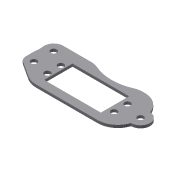
# Autodesk Inventor part: Adapter
Saved by Autodesk Inventor 2015 (Build 190159000, 159)
## iProperties
Created: 2015-02-12
Part Number: Adapter
Material: Generisch
Document SubType Name: Modeling
Designer: Luki
Density: 1 g/cm^3
Appearance: Vorgabe
Author: Luki
Autodesk Inventor part; units mm, degrees
ref_plane "YZ Plane" through (0, 0, 0) normal (1, 0, 0) x (0, 1, 0)
ref_plane "XZ Plane" through (0, 0, 0) normal (0, 1, 0) x (-1, 0, 0)
ref_plane "XY Plane" through (0, 0, 0) normal (0, 0, 1) x (1, 0, 0)
sketch "Skizze1" plane through (0, 0, 0) normal (0, 0, 1) x (1, 0, 0)
  line L0 (0, 78) -> (0, -13) projected
  line L1 (-15, 0) -> (90, 0) projected
  line L2 (0, 0) -> (75, 0)
  line L3 (75, 0) -> (75, 35)
  line L4 (75, 35) -> (0, 35)
  line L5 (0, 35) -> (0, 0)
  arc A0 (24, 35) -> (56, 35) centre (40, 65) ccw
  dimension "d0" = 75
  dimension "d1" = 35
  dimension "d3" = 35
  dimension "d4" = 30
  dimension "d6" = 34
  constraints: 8 end point, 2 parallel, 2 point on circle, 2 point on line, 1 centre point, 1 horizontal, 1 perpendicular
  measures "d0" distance between parallel lines of L3 L0
  measures "d1" distance between parallel lines of L4 L1
  measures "d3" distance from line of L3 A0.centre
  measures "d4" distance from line of L4 A0.centre
  measures "d6" radius of A0
extrude "Extrusion1" add sketch "Skizze1" along normal blind 2 contours L4 A0 L3 L1 L0
sketch "Skizze2" plane through (0, 0, 2) normal (0, 0, 1) x (1, 0, 0)
  line L0 (36, 6) -> (57, 6)
  line L1 (57, 6) -> (57, 27)
  line L2 (57, 27) -> (36, 27)
  line L3 (36, 27) -> (36, 6)
  line L4 (36, 6) -> (57, 27) construction
  line L5 (57, 6) -> (36, 27) construction
  line L6 (57, 27) -> (15, 27)
  line L7 (15, 27) -> (15, 6)
  line L8 (15, 6) -> (57, 6)
  line L9 (57, 6) -> (57, 27)
  line L10 (75, 0) -> (75, 35) projected
  line L11 (24, 35) -> (0, 35) projected
  circle A0 centre (61.35, 21.5) radius 2.25
  circle A1 centre (61.35, 11.5) radius 2.25
  circle A2 centre (11.85, 11.5) radius 2.25
  circle A3 centre (11.85, 21.5) radius 2.25
  point P0 (0, 0)
  point P1 (46.5, 16.5)
  dimension "d9" = 21
  dimension "d10" = 21
  dimension "d11" = 42
  dimension "d12" = 0
  dimension "d13" = 18
  dimension "d14" = 8
  dimension "d15" = 4.5
  dimension "d16" = 4.5
  dimension "d17" = 4.5
  dimension "d18" = 4.5
  dimension "d19" = 14.85
  dimension "d20" = 5
  dimension "d21" = 5
  dimension "d22" = 14.85
  dimension "d23" = 34.65
  dimension "d24" = 34.65
  dimension "d27" = 5
  dimension "d28" = 5
  constraints: 20 end point, 4 centre point, 4 parallel, 2 horizontal, 2 midpoint, 2 perpendicular
  measures "d9" distance between parallel lines of L0 L2
  measures "d10" distance between parallel lines of L3 L1
  measures "d11" distance between parallel lines of L1 L7
  measures "d12" distance between parallel lines of L0 L8
  measures "d13" distance between parallel lines of L10 L1
  measures "d14" distance between parallel lines of L11 L6
  measures "d15" diameter of A0
  measures "d16" diameter of A1
  measures "d17" diameter of A3
  measures "d18" diameter of A2
  measures "d19" horizontal distance of point (46.5, 16.5) A1.centre
  measures "d20" vertical distance of point (46.5, 16.5) A1.centre
  measures "d21" vertical distance of point (46.5, 16.5) A0.centre
  measures "d22" horizontal distance of point (46.5, 16.5) A0.centre
  measures "d23" horizontal distance of point (46.5, 16.5) A3.centre
  measures "d24" horizontal distance of point (46.5, 16.5) A2.centre
  measures "d27" vertical distance of point (46.5, 16.5) A2.centre
  measures "d28" vertical distance of point (46.5, 16.5) A3.centre
extrude "Extrusion2" cut sketch "Skizze2" against normal blind 2
sketch "Skizze3" plane through (0, 0, 2) normal (0, 0, 1) x (1, 0, 0)
  circle A0 centre (11.85, 21.5) radius 2.25 projected
  circle A1 centre (61.35, 11.5) radius 2.25 projected
  circle A2 centre (61.35, 21.5) radius 2.25 projected
  circle A3 centre (11.85, 11.5) radius 2.25 projected
  line L0 (15, 27) -> (15, 6) projected
  line L1 (15, 6) -> (57, 6) projected
  line L2 (57, 6) -> (57, 27) projected
  line L3 (57, 27) -> (15, 27) projected
  line L4 (0, 0) -> (0, 35) projected
  line L5 (0, 35) -> (24, 35) projected
  arc A4 (24, 35) -> (56, 35) centre (40, 65) ccw projected
  line L6 (56, 35) -> (75, 35) projected
  line L7 (75, 35) -> (75, 0) projected
  line L8 (75, 0) -> (0, 0) projected
  line L9 (75, 0) -> (75, 35) projected
  circle A5 centre (75, 17.5) radius 7
  line L10 (75, 0) -> (75, 35) projected
  dimension "d31" = 14
  dimension "d32" = 35
  dimension "d33" = 17.5
  constraints: 2 midpoint, 1 centre point
  measures "d31" diameter of A5
  measures "d32" distance between parallel lines of L8 L6
  measures "d33" distance from line of L8 A5.centre
extrude "Extrusion3" add sketch "Skizze3" against normal blind 2 contours A5 L7 | L7 A5
sketch "Skizze4" plane through (0, 0, 2) normal (0, 0, 1) x (1, 0, 0)
  circle A0 centre (11.85, 21.5) radius 2.25 projected
  circle A1 centre (61.35, 11.5) radius 2.25 projected
  circle A2 centre (61.35, 21.5) radius 2.25 projected
  circle A3 centre (11.85, 11.5) radius 2.25 projected
  line L0 (15, 27) -> (15, 6) projected
  line L1 (15, 6) -> (57, 6) projected
  line L2 (57, 6) -> (57, 27) projected
  line L3 (57, 27) -> (15, 27) projected
  line L4 (0, 0) -> (0, 35) projected
  line L5 (0, 35) -> (24, 35) projected
  arc A4 (24, 35) -> (56, 35) centre (40, 65) ccw projected
  line L6 (56, 35) -> (75, 35) projected
  line L7 (75, 35) -> (75, 24.5) projected
  arc A5 (75, 10.5) -> (75, 24.5) centre (75, 17.5) ccw projected
  line L8 (75, 10.5) -> (75, 0) projected
  line L9 (75, 0) -> (0, 0) projected
  circle A6 centre (75, 17.5) radius 2.25
  dimension "d36" = 4.5
  constraints: 1 centre point, 1 coincident
  measures "d36" diameter of A6
extrude "Extrusion4" cut sketch "Skizze4" against normal blind 2 contours A6
fillet "Rundung1" radius 15 1 edges at (0, 0, 1)
sketch "Skizze5" plane through (0, 0, 2) normal (0, 0, 1) x (1, 0, 0)
  line L0 (0, 35) -> (0, 15) projected
  circle A0 centre (0, 28) radius 7
  circle A1 centre (75, 17.5) radius 2.25 projected
  arc A2 (75, 10.5) -> (75, 24.5) centre (75, 17.5) ccw projected
  line L1 (75, 10.5) -> (75, 0) projected
  line L2 (75, 0) -> (15, 0) projected
  arc A3 (0, 15) -> (15, 0) centre (15, 15) ccw projected
  line L3 (0, 15) -> (0, 35) projected
  line L4 (0, 35) -> (24, 35) projected
  arc A4 (24, 35) -> (56, 35) centre (40, 65) ccw projected
  line L5 (56, 35) -> (75, 35) projected
  line L6 (75, 35) -> (75, 24.5) projected
  circle A5 centre (11.85, 21.5) radius 2.25 projected
  circle A6 centre (61.35, 11.5) radius 2.25 projected
  circle A7 centre (61.35, 21.5) radius 2.25 projected
  circle A8 centre (11.85, 11.5) radius 2.25 projected
  line L7 (15, 27) -> (15, 6) projected
  line L8 (15, 6) -> (57, 6) projected
  line L9 (57, 6) -> (57, 27) projected
  line L10 (57, 27) -> (15, 27) projected
  circle A9 centre (0, 21) radius 7
  point P0 (0, 0)
  dimension "d40" = 14
  dimension "d46" = 14
  constraints: 2 centre point, 2 point on circle, 1 point on line
  measures "d40" diameter of A0
  measures "d46" diameter of A9
extrude "Extrusion5" add sketch "Skizze5" against normal blind 2 contours A0 A9 L0 | L0 A9 A0 | A9 A0 L0 | L0 A0 A9 | A0 L0 A3 A9 | A0 A9 A3 L0
sketch "Skizze6" plane through (0, 0, 2) normal (0, 0, 1) x (1, 0, 0)
  circle A0 centre (75, 17.5) radius 2.25 projected
  arc A1 (75, 10.5) -> (75, 24.5) centre (75, 17.5) ccw projected
  line L0 (75, 10.5) -> (75, 0) projected
  line L1 (75, 0) -> (15, 0) projected
  line L2 (0, 35) -> (24, 35) projected
  arc A2 (24, 35) -> (56, 35) centre (40, 65) ccw projected
  line L3 (56, 35) -> (75, 35) projected
  line L4 (75, 35) -> (75, 24.5) projected
  circle A3 centre (11.85, 21.5) radius 2.25 projected
  circle A4 centre (61.35, 11.5) radius 2.25 projected
  circle A5 centre (61.35, 21.5) radius 2.25 projected
  circle A6 centre (11.85, 11.5) radius 2.25 projected
  line L5 (15, 27) -> (15, 6) projected
  line L6 (15, 6) -> (57, 6) projected
  line L7 (57, 6) -> (57, 27) projected
  line L8 (57, 27) -> (15, 27) projected
  circle A7 centre (0, 28) radius 2.25
  circle A8 centre (75, 17.5) radius 75.7314
  circle A9 centre (-0.7298, 18) radius 7
  arc A10 (0.0334, 14.0001) -> (15, 0) centre (15, 15) ccw projected
  arc A11 (-6.0622, 24.5) -> (0.0334, 14.0001) centre (0, 21) ccw projected
  arc A12 (0, 35) -> (-6.0622, 24.5) centre (0, 28) ccw projected
  point P0 (0, 0)
  point P1 (0, 21)
  dimension "d43" = 4.5
  dimension "d47" = 14
  dimension "d48" = 3
  constraints: 3 centre point, 2 coincident, 2 point on circle
  measures "d43" diameter of A7
  measures "d47" diameter of A9
  measures "d48" vertical distance of A9.centre point (0, 21)
extrude "Extrusion6" cut sketch "Skizze6" against normal blind 2 contours A8 A7 | A7 A8
fillet "Rundung2" radius 15 2 edges at (-6.0622, 24.5, 1) (0.0334, 14.0001, 1)
sketch "Skizze7" plane through (0, 0, 2) normal (0, 0, 1) x (1, 0, 0)
  circle A0 centre (0, 28) radius 2.25 projected
  circle A1 centre (75, 17.5) radius 2.25 projected
  arc A2 (75, 10.5) -> (75, 24.5) centre (75, 17.5) ccw projected
  line L0 (75, 10.5) -> (75, 0) projected
  line L1 (75, 0) -> (15, 0) projected
  arc A3 (1.286, 8.9233) -> (15, 0) centre (15, 15) ccw projected
  arc A4 (1.286, 8.9233) -> (-3.9544, 15.2239) centre (-12.428, 2.8466) ccw projected
  arc A5 (-6.9108, 22.1136) -> (-3.9544, 15.2239) centre (0, 21) ccw projected
  arc A6 (-6.9108, 22.1136) -> (-6.9108, 26.8864) centre (-21.7198, 24.5) ccw projected
  arc A7 (0, 35) -> (-6.9108, 26.8864) centre (0, 28) ccw projected
  line L2 (0, 35) -> (24, 35) projected
  arc A8 (24, 35) -> (56, 35) centre (40, 65) ccw projected
  line L3 (56, 35) -> (75, 35) projected
  line L4 (75, 35) -> (75, 24.5) projected
  circle A9 centre (11.85, 21.5) radius 2.25 projected
  circle A10 centre (61.35, 11.5) radius 2.25 projected
  circle A11 centre (61.35, 21.5) radius 2.25 projected
  circle A12 centre (11.85, 11.5) radius 2.25 projected
  line L5 (15, 27) -> (15, 6) projected
  line L6 (15, 6) -> (57, 6) projected
  line L7 (57, 6) -> (57, 27) projected
  line L8 (57, 27) -> (15, 27) projected
  arc A13 (75, 10.5) -> (75, 24.5) centre (75, 17.5) ccw projected
  circle A14 centre (75, 17.5) radius 75.7314
  circle A15 centre (-0.7166, 19) radius 2.25
  point P0 (0, 0)
  dimension "d50" = 9
  dimension "d51" = 4.5
  constraints: 2 centre point, 2 point on circle, 1 coincident
  measures "d50" vertical distance of A0.centre A15.centre
  measures "d51" diameter of A15
extrude "Extrusion7" cut sketch "Skizze7" against normal blind 2 contours A15 A14 | A14 A15
fillet "Rundung3" radius 15 4 edges at (75, 35, 1) (56, 35, 1) (24, 35, 1) (75, 0, 1)
sketch "Skizze8" plane through (0, 0, 2) normal (0, 0, 1) x (1, 0, 0)
  circle A0 centre (-0.7166, 19) radius 2.25 projected
  arc A1 (1.286, 8.9233) -> (-3.9544, 15.2239) centre (-12.428, 2.8466) ccw projected
  arc A2 (-6.9108, 22.1136) -> (-3.9544, 15.2239) centre (0, 21) ccw projected
  arc A3 (-6.9108, 22.1136) -> (-6.9108, 26.8864) centre (-21.7198, 24.5) ccw projected
  arc A4 (0, 35) -> (-6.9108, 26.8864) centre (0, 28) ccw projected
  line L0 (0, 35) -> (20.6093, 35) projected
  arc A5 (26.5452, 33.7755) -> (20.6093, 35) centre (20.6093, 20) ccw projected
  arc A6 (26.5452, 33.7755) -> (53.4548, 33.7755) centre (40, 65) ccw projected
  arc A7 (59.3907, 35) -> (53.4548, 33.7755) centre (59.3907, 20) ccw projected
  line L1 (59.3907, 35) -> (60.6909, 35) projected
  arc A8 (75, 24.5) -> (60.6909, 35) centre (60.6909, 20) ccw projected
  arc A9 (75, 10.5) -> (75, 24.5) centre (75, 17.5) ccw projected
  arc A10 (60.6909, 0) -> (75, 10.5) centre (60.6909, 15) ccw projected
  line L2 (60.6909, 0) -> (15, 0) projected
  arc A11 (1.286, 8.9233) -> (15, 0) centre (15, 15) ccw projected
  circle A12 centre (0, 28) radius 2.25 projected
  circle A13 centre (75, 17.5) radius 2.25 projected
  circle A14 centre (11.85, 21.5) radius 2.25 projected
  circle A15 centre (61.35, 11.5) radius 2.25 projected
  circle A16 centre (61.35, 21.5) radius 2.25 projected
  circle A17 centre (11.85, 11.5) radius 2.25 projected
  line L3 (15, 27) -> (15, 6) projected
  line L4 (15, 6) -> (57, 6) projected
  line L5 (57, 6) -> (57, 27) projected
  line L6 (57, 27) -> (15, 27) projected
  circle A18 centre (75, 17.5) radius 2.25 projected
  circle A19 centre (75, 17.5) radius 82.0816
  line L7 (-6.8487, 11.3205) -> (6.8192, 2.4272)
  arc A20 (1.286, 8.9233) -> (15, 0) centre (15, 15) ccw projected
  line L8 (6.8192, 2.4272) -> (-0.8956, 15)
  line L9 (-0.8956, 15) -> (-5.8598, 18.2396)
  line L10 (-5.8598, 18.2396) -> (-6.9924, 21.3263)
  arc A21 (-6.9108, 22.1136) -> (-3.9544, 15.2239) centre (0, 21) ccw projected
  point P0 (0, 0)
  constraints: 8 end point, 5 point on circle, 2 tangent, 1 centre point, 1 coincident
extrude "Extrusion8" add sketch "Skizze8" against normal blind 2 contours A11 L7 A19 A2 A1 | A1 A2 L10 L9 L8 A11
fillet "Rundung4" radius 5 1 edges at (-6.8487, 11.3205, 1)
sketch "Skizze9" plane through (0, 0, 2) normal (0, 0, 1) x (1, 0, 0)
  arc A0 (26.5452, 33.7755) -> (20.6093, 35) centre (20.6093, 20) ccw projected
  arc A1 (26.5452, 33.7755) -> (53.4548, 33.7755) centre (40, 65) ccw projected
  arc A2 (59.3907, 35) -> (53.4548, 33.7755) centre (59.3907, 20) ccw projected
  line L0 (59.3907, 35) -> (60.6909, 35) projected
  arc A3 (75, 24.5) -> (60.6909, 35) centre (60.6909, 20) ccw projected
  arc A4 (75, 10.5) -> (75, 24.5) centre (75, 17.5) ccw projected
  arc A5 (60.6909, 0) -> (75, 10.5) centre (60.6909, 15) ccw projected
  line L1 (60.6909, 0) -> (15, 0) projected
  arc A6 (6.8192, 2.4272) -> (15, 0) centre (15, 15) ccw projected
  line L2 (6.8192, 2.4272) -> (-4.7351, 9.9453) projected
  arc A7 (-7.0034, 13.918) -> (-4.7351, 9.9453) centre (-2.0082, 14.1362) ccw projected
  arc A8 (-6.9924, 21.3263) -> (-7.0034, 13.918) centre (75, 17.5) ccw projected
  arc A9 (-6.9108, 22.1136) -> (-6.9924, 21.3263) centre (0, 21) ccw projected
  arc A10 (-6.9108, 22.1136) -> (-6.9108, 26.8864) centre (-21.7198, 24.5) ccw projected
  arc A11 (0, 35) -> (-6.9108, 26.8864) centre (0, 28) ccw projected
  line L3 (0, 35) -> (20.6093, 35) projected
  circle A12 centre (-0.7166, 19) radius 2.25 projected
  circle A13 centre (0, 28) radius 2.25 projected
  circle A14 centre (75, 17.5) radius 2.25 projected
  circle A15 centre (11.85, 21.5) radius 2.25 projected
  circle A16 centre (61.35, 11.5) radius 2.25 projected
  circle A17 centre (61.35, 21.5) radius 2.25 projected
  circle A18 centre (11.85, 11.5) radius 2.25 projected
  line L4 (15, 27) -> (15, 6) projected
  line L5 (15, 6) -> (57, 6) projected
  line L6 (57, 6) -> (57, 27) projected
  line L7 (57, 27) -> (15, 27) projected
  point P0 (0, 0)
extrude "Extrusion9" add sketch "Skizze9" against normal up to surface (2 mm away) contours A12
sketch "Skizze10" plane through (0, 0, 2) normal (0, 0, 1) x (1, 0, 0)
  arc A0 (26.5452, 33.7755) -> (20.6093, 35) centre (20.6093, 20) ccw projected
  arc A1 (26.5452, 33.7755) -> (53.4548, 33.7755) centre (40, 65) ccw projected
  arc A2 (59.3907, 35) -> (53.4548, 33.7755) centre (59.3907, 20) ccw projected
  line L0 (59.3907, 35) -> (60.6909, 35) projected
  arc A3 (75, 24.5) -> (60.6909, 35) centre (60.6909, 20) ccw projected
  arc A4 (75, 10.5) -> (75, 24.5) centre (75, 17.5) ccw projected
  arc A5 (60.6909, 0) -> (75, 10.5) centre (60.6909, 15) ccw projected
  line L1 (60.6909, 0) -> (15, 0) projected
  arc A6 (6.8192, 2.4272) -> (15, 0) centre (15, 15) ccw projected
  line L2 (6.8192, 2.4272) -> (-4.7351, 9.9453) projected
  arc A7 (-7.0034, 13.918) -> (-4.7351, 9.9453) centre (-2.0082, 14.1362) ccw projected
  arc A8 (-6.9924, 21.3263) -> (-7.0034, 13.918) centre (75, 17.5) ccw projected
  arc A9 (-6.9108, 22.1136) -> (-6.9924, 21.3263) centre (0, 21) ccw projected
  arc A10 (-6.9108, 22.1136) -> (-6.9108, 26.8864) centre (-21.7198, 24.5) ccw projected
  arc A11 (0, 35) -> (-6.9108, 26.8864) centre (0, 28) ccw projected
  line L3 (0, 35) -> (20.6093, 35) projected
  circle A12 centre (0, 28) radius 2.25 projected
  circle A13 centre (75, 17.5) radius 2.25 projected
  circle A14 centre (11.85, 21.5) radius 2.25 projected
  circle A15 centre (61.35, 11.5) radius 2.25 projected
  circle A16 centre (61.35, 21.5) radius 2.25 projected
  circle A17 centre (11.85, 11.5) radius 2.25 projected
  line L4 (15, 27) -> (15, 6) projected
  line L5 (15, 6) -> (57, 6) projected
  line L6 (57, 6) -> (57, 27) projected
  line L7 (57, 27) -> (15, 27) projected
  circle A18 centre (75, 17.5) radius 75.7314
  circle A19 centre (-0.6505, 14) radius 2.25
  point P0 (0, 0)
  dimension "d60" = 14
  dimension "d61" = 4.5
  constraints: 2 centre point, 2 point on circle, 1 coincident
  measures "d60" vertical distance of A11.centre A19.centre
  measures "d61" diameter of A19
extrude "Extrusion10" cut sketch "Skizze10" against normal blind 2 contours A19 A18 | A18 A19
equation "\"d16\" = d15"
equation "\"d17\" = d15"
equation "\"d18\" = d17"
equation "\"d21\" = d20"
equation "\"d22\" = d19"
equation "\"d24\" = d23"
equation "\"d28\" = d27"
equation "\"d33\" = 0.5 * d32"
